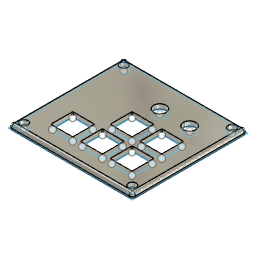
top (Autodesk Fusion 360 design; units mm, degrees)
part number: 2026-08-13-23-21-25-197
Autodesk Fusion 360 part; units mm, degrees
sketch "sketch 480" plane through (0, 0, 10) normal (0, 0, 1) x (-1, 0, 0)
  line L0 (-127.5, 108.6) -> (-127.5, 121.6)
  line L1 (-127.5, 108.6) -> (-127.5, 121.6)
  arc A0 (-127.5, 121.6) -> (-127, 122.1) centre (-127, 121.6) cw
  arc A1 (-127.5, 121.6) -> (-127, 122.1) centre (-127, 121.6) cw
  line L2 (-127, 122.1) -> (-114, 122.1)
  line L3 (-127, 122.1) -> (-114, 122.1)
  arc A2 (-114, 122.1) -> (-113.5, 121.6) centre (-114, 121.6) cw
  arc A3 (-114, 122.1) -> (-113.5, 121.6) centre (-114, 121.6) cw
  line L4 (-113.5, 121.6) -> (-113.5, 108.6)
  line L5 (-113.5, 121.6) -> (-113.5, 108.6)
  arc A4 (-113.5, 108.6) -> (-114, 108.1) centre (-114, 108.6) cw
  arc A5 (-113.5, 108.6) -> (-114, 108.1) centre (-114, 108.6) cw
  line L6 (-114, 108.1) -> (-127, 108.1)
  line L7 (-114, 108.1) -> (-127, 108.1)
  arc A6 (-127, 108.1) -> (-127.5, 108.6) centre (-127, 108.6) cw
  arc A7 (-127, 108.1) -> (-127.5, 108.6) centre (-127, 108.6) cw
  arc A8 (-146.55, 140.65) -> (-146.05, 141.15) centre (-146.05, 140.65) cw
  arc A9 (-146.55, 140.65) -> (-146.05, 141.15) centre (-146.05, 140.65) cw
  line L8 (-146.05, 141.15) -> (-133.05, 141.15)
  line L9 (-146.05, 141.15) -> (-133.05, 141.15)
  arc A10 (-133.05, 141.15) -> (-132.55, 140.65) centre (-133.05, 140.65) cw
  arc A11 (-133.05, 141.15) -> (-132.55, 140.65) centre (-133.05, 140.65) cw
  line L10 (-132.55, 140.65) -> (-132.55, 127.65)
  line L11 (-132.55, 140.65) -> (-132.55, 127.65)
  arc A12 (-132.55, 127.65) -> (-133.05, 127.15) centre (-133.05, 127.65) cw
  arc A13 (-132.55, 127.65) -> (-133.05, 127.15) centre (-133.05, 127.65) cw
  line L12 (-133.05, 127.15) -> (-146.05, 127.15)
  line L13 (-133.05, 127.15) -> (-146.05, 127.15)
  arc A14 (-146.05, 127.15) -> (-146.55, 127.65) centre (-146.05, 127.65) cw
  arc A15 (-146.05, 127.15) -> (-146.55, 127.65) centre (-146.05, 127.65) cw
  line L14 (-146.55, 127.65) -> (-146.55, 140.65)
  line L15 (-146.55, 127.65) -> (-146.55, 140.65)
  circle A16 centre (-154.5512, 85) radius 2.5
  circle A17 centre (-120.8661, 97.6058) radius 4
  circle A18 centre (-85.0512, 85) radius 2.5
  arc A19 (-108.45, 140.65) -> (-107.95, 141.15) centre (-107.95, 140.65) cw
  arc A20 (-108.45, 140.65) -> (-107.95, 141.15) centre (-107.95, 140.65) cw
  line L16 (-107.95, 141.15) -> (-94.95, 141.15)
  line L17 (-107.95, 141.15) -> (-94.95, 141.15)
  arc A21 (-94.95, 141.15) -> (-94.45, 140.65) centre (-94.95, 140.65) cw
  arc A22 (-94.95, 141.15) -> (-94.45, 140.65) centre (-94.95, 140.65) cw
  line L18 (-94.45, 140.65) -> (-94.45, 127.65)
  line L19 (-94.45, 140.65) -> (-94.45, 127.65)
  arc A23 (-94.45, 127.65) -> (-94.95, 127.15) centre (-94.95, 127.65) cw
  arc A24 (-94.45, 127.65) -> (-94.95, 127.15) centre (-94.95, 127.65) cw
  line L20 (-94.95, 127.15) -> (-107.95, 127.15)
  line L21 (-94.95, 127.15) -> (-107.95, 127.15)
  arc A25 (-107.95, 127.15) -> (-108.45, 127.65) centre (-107.95, 127.65) cw
  arc A26 (-107.95, 127.15) -> (-108.45, 127.65) centre (-107.95, 127.65) cw
  line L22 (-108.45, 127.65) -> (-108.45, 140.65)
  line L23 (-108.45, 127.65) -> (-108.45, 140.65)
  arc A27 (-127.5, 140.65) -> (-127, 141.15) centre (-127, 140.65) cw
  arc A28 (-127.5, 140.65) -> (-127, 141.15) centre (-127, 140.65) cw
  line L24 (-127, 141.15) -> (-114, 141.15)
  line L25 (-127, 141.15) -> (-114, 141.15)
  arc A29 (-114, 141.15) -> (-113.5, 140.65) centre (-114, 140.65) cw
  arc A30 (-114, 141.15) -> (-113.5, 140.65) centre (-114, 140.65) cw
  line L26 (-113.5, 140.65) -> (-113.5, 127.65)
  line L27 (-113.5, 140.65) -> (-113.5, 127.65)
  arc A31 (-113.5, 127.65) -> (-114, 127.15) centre (-114, 127.65) cw
  arc A32 (-113.5, 127.65) -> (-114, 127.15) centre (-114, 127.65) cw
  line L28 (-114, 127.15) -> (-127, 127.15)
  line L29 (-114, 127.15) -> (-127, 127.15)
  arc A33 (-127, 127.15) -> (-127.5, 127.65) centre (-127, 127.65) cw
  arc A34 (-127, 127.15) -> (-127.5, 127.65) centre (-127, 127.65) cw
  line L30 (-127.5, 127.65) -> (-127.5, 140.65)
  line L31 (-127.5, 127.65) -> (-127.5, 140.65)
  arc A35 (-146.55, 121.6) -> (-146.05, 122.1) centre (-146.05, 121.6) cw
  arc A36 (-146.55, 121.6) -> (-146.05, 122.1) centre (-146.05, 121.6) cw
  line L32 (-146.05, 122.1) -> (-133.05, 122.1)
  line L33 (-146.05, 122.1) -> (-133.05, 122.1)
  arc A37 (-133.05, 122.1) -> (-132.55, 121.6) centre (-133.05, 121.6) cw
  arc A38 (-133.05, 122.1) -> (-132.55, 121.6) centre (-133.05, 121.6) cw
  line L34 (-132.55, 121.6) -> (-132.55, 108.6)
  line L35 (-132.55, 121.6) -> (-132.55, 108.6)
  arc A39 (-132.55, 108.6) -> (-133.05, 108.1) centre (-133.05, 108.6) cw
  arc A40 (-132.55, 108.6) -> (-133.05, 108.1) centre (-133.05, 108.6) cw
  line L36 (-133.05, 108.1) -> (-146.05, 108.1)
  line L37 (-133.05, 108.1) -> (-146.05, 108.1)
  arc A41 (-146.05, 108.1) -> (-146.55, 108.6) centre (-146.05, 108.6) cw
  arc A42 (-146.05, 108.1) -> (-146.55, 108.6) centre (-146.05, 108.6) cw
  line L38 (-146.55, 108.6) -> (-146.55, 121.6)
  line L39 (-146.55, 108.6) -> (-146.55, 121.6)
  circle A43 centre (-154.5512, 149) radius 2.5
  line L40 (-159.5512, 154) -> (-159.5512, 80)
  line L41 (-159.5512, 80) -> (-80.0512, 80)
  line L42 (-80.0512, 80) -> (-80.0512, 154)
  line L43 (-80.0512, 154) -> (-159.5512, 154)
  circle A44 centre (-85.0512, 149) radius 2.5
  circle A45 centre (-139.9661, 97.6058) radius 4
extrude "Extrude1" add sketch "sketch 480" along normal blind 3
fillet "Fillet1" radius 2 8 edges at (159.5512, -154, 11.5) (159.5512, -117, 13) (119.8012, -154, 13) (119.8012, -80, 13) (159.5512, -80, 11.5) (80.0512, -117, 13) (80.0512, -154, 11.5) (80.0512, -80, 11.5)
